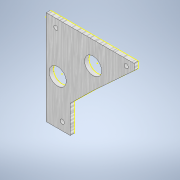
# Autodesk Inventor part: アームギアフレーム最内
Saved by Autodesk Inventor 2020.2 (Build 242310000, 310)
## iProperties
Created: 2020-02-29
Part Number: アームギアフレーム最内
Material: アルミニウム 7075
Document SubType Name: Modeling
Designer: aoyam
Density: 2.81 g/cm^3
Appearance: サテン - ブラシ仕上げ 重厚
Author: aoyam
Autodesk Inventor part; units mm, degrees
ref_plane "YZ Plane" through (0, 0, 0) normal (1, 0, 0) x (0, 1, 0)
ref_plane "XZ Plane" through (0, 0, 0) normal (0, 1, 0) x (-1, 0, 0)
sketch "ギア線図" plane through (0, 0, 0) normal (0, 0, 1) x (1, 0, 0)
  circle A0 centre (11.2246, -29.111) radius 11.1
  circle A1 centre (54.569, -27.2294) radius 20.05
  circle A2 centre (54.569, -27.2294) radius 4
  circle A3 centre (36.0807, -10.2532) radius 11.1
  circle A4 centre (39.569, -43.72) radius 2.05
  circle A5 centre (69.569, -43.72) radius 2.05
  circle A6 centre (72.4026, -13.8541) radius 2.05
  circle A7 centre (39.569, -43.72) radius 15
  circle A8 centre (69.569, -43.72) radius 15
  circle A9 centre (72.4026, -13.8541) radius 15
  circle A10 centre (54.569, -27.2294) radius 5.5 construction
  circle A11 centre (11.2246, -29.111) radius 13 construction
  circle A12 centre (54.569, -27.2294) radius 20.5 construction
  circle A13 centre (36.0807, -10.2532) radius 20.55
  circle A14 centre (36.0807, -10.2532) radius 21.5 construction
  circle A15 centre (36.0807, -10.2532) radius 13 construction
  circle A16 centre (39.569, -43.72) radius 2.5 construction
  circle A17 centre (69.569, -43.72) radius 2.5 construction
  circle A18 centre (72.4026, -13.8541) radius 2.5 construction
  circle A19 centre (11.2246, -29.111) radius 20.1
  circle A20 centre (11.2246, -29.111) radius 22 construction
  line L0 (39.569, -43.72) -> (69.569, -43.72)
  circle A21 centre (0, 0) radius 20.1
  circle A22 centre (0, 0) radius 22 construction
  circle A23 centre (39.569, -43.72) radius 9.5 construction
  circle A24 centre (69.569, -43.72) radius 9.5 construction
  circle A25 centre (72.4026, -13.8541) radius 9.5 construction
  line L1 (39.569, -43.72) -> (33.651, -38.3369)
  line L2 (39.569, -43.72) -> (54.569, -27.2294)
  circle A26 centre (33.651, -38.3369) radius 2.25
  circle A27 centre (54.569, -27.2294) radius 4.55
  point P0 (58.2233, -20.0465)
  point P1 (42.0436, -35)
  point P2 (21.5995, 15.2696)
  point P3 (38.2329, 5.9161)
  point P4 (24.1755, 8.4229)
  point P5 (21.6039, 15.1272)
  point P6 (23.3458, 16.3469)
  point P7 (23.3177, 16.3886)
  dimension "d7" = 22.2
  dimension "d8" = 40.1
  dimension "d9" = 8
  dimension "d11" = 22.2
  dimension "d12" = 4.1
  dimension "d13" = 4.1
  dimension "d14" = 4.1
  dimension "d15" = 30
  dimension "d16" = 30
  dimension "d17" = 30
  dimension "d18" = 11
  dimension "d21" = 26
  dimension "d29" = 41
  dimension "d39" = 22.2921
  dimension "d40" = 22.2921
  dimension "d41" = 22.2921
  dimension "d43" = 41.1
  dimension "d44" = 43
  dimension "d45" = 26
  dimension "d46" = 5
  dimension "d47" = 5
  dimension "d48" = 5
  dimension "d49" = 40.2
  dimension "d50" = 44
  dimension "d53" = 40.2
  dimension "d55" = 44
  dimension "d58" = 19
  dimension "d59" = 19
  dimension "d60" = 19
  dimension "d86" = 8
  dimension "d87" = 4.5
  constraints: 28 centre point, 17 coincident, 7 tangent, 6 end point, 3 concentric, 2 horizontal, 1 perpendicular, 1 other
  measures "d7" diameter of A0
  measures "d8" diameter of A1
  measures "d9" diameter of A2
  measures "d11" diameter of A3
  measures "d12" diameter of A4
  measures "d13" diameter of A5
  measures "d14" diameter of A6
  measures "d15" diameter of A7
  measures "d16" diameter of A8
  measures "d17" diameter of A9
  measures "d18" diameter of A10
  measures "d21" diameter of A11
  measures "d29" diameter of A12
  measures "d39" distance of A4.centre A1.centre
  measures "d40" distance of A5.centre A1.centre
  measures "d41" distance of A6.centre A1.centre
  measures "d43" diameter of A13
  measures "d44" diameter of A14
  measures "d45" diameter of A15
  measures "d46" diameter of A16
  measures "d47" diameter of A17
  measures "d48" diameter of A18
  measures "d49" diameter of A19
  measures "d50" diameter of A20
  measures "d53" diameter of A21
  measures "d55" diameter of A22
  measures "d58" diameter of A23
  measures "d59" diameter of A24
  measures "d60" diameter of A25
  measures "d86" distance of L1.start L1.end
  measures "d87" diameter of A26
sketch "スケッチ3" plane through (0, 0, 0) normal (0, 0, 1) x (1, 0, 0)
  circle A0 centre (54.569, -27.2294) radius 20.05 construction
  circle A1 centre (39.569, -43.72) radius 2.05 construction
  circle A2 centre (69.569, -43.72) radius 2.05 construction
  circle A3 centre (72.4026, -13.8541) radius 2.05 construction
  circle A4 centre (39.569, -43.72) radius 15 construction
  circle A5 centre (69.569, -43.72) radius 15 construction
  circle A6 centre (72.4026, -13.8541) radius 15 construction
  line L0 (39.569, -43.72) -> (45.487, -49.103)
  line L1 (45.487, -49.103) -> (39.569, -43.72)
  line L2 (39.569, -43.72) -> (33.651, -38.3369)
  line L3 (39.569, -43.72) -> (41.0777, -42.0614)
  circle A7 centre (33.651, -38.3369) radius 1.3
  circle A8 centre (45.487, -49.103) radius 1.3
  line L4 (69.569, -43.72) -> (68.0603, -42.0614)
  line L5 (69.569, -43.72) -> (75.487, -38.3369)
  line L6 (69.569, -43.72) -> (63.651, -49.103)
  circle A9 centre (63.651, -49.103) radius 1.3
  circle A10 centre (75.487, -38.3369) radius 1.3
  line L7 (72.4026, -13.8541) -> (70.609, -15.1993)
  line L8 (67.6026, -7.4541) -> (72.4026, -13.8541)
  line L9 (72.4026, -13.8541) -> (77.2027, -20.2541)
  circle A11 centre (67.6026, -7.4541) radius 1.3
  circle A12 centre (77.2027, -20.2541) radius 1.3
  circle A13 centre (39.569, -43.72) radius 5
  circle A14 centre (69.569, -43.72) radius 5
  circle A15 centre (72.4026, -13.8541) radius 5
  circle A16 centre (54.569, -27.2294) radius 4
  circle A17 centre (36.0807, -10.2532) radius 11.1 construction
  line L10 (87.4026, -58.72) -> (21.3486, -58.72)
  line L11 (87.4026, 3.1749) -> (87.4026, -58.72)
  circle A18 centre (36.0807, -10.2532) radius 6
  circle A19 centre (23.1948, 12.8161) radius 1.5
  circle A20 centre (59.3303, 1.1874) radius 1.5
  circle A21 centre (11.2246, -29.111) radius 6
  circle A22 centre (14.4482, -54.9706) radius 1.5
  line L12 (87.4026, 3.1749) -> (31.1389, 3.1749)
  line L13 (31.1389, 3.1749) -> (25.7575, 16.2256)
  line L14 (26.6296, -46.3454) -> (10.2913, -53.0824)
  line L15 (10.2913, -53.0824) -> (10.2913, -58.72)
  line L16 (10.2913, -58.72) -> (21.3486, -58.72)
  line L17 (26.6296, -46.3454) -> (26.6296, -10.2532)
  line L18 (26.6296, -10.2532) -> (18.7982, 13.9762)
  line L19 (18.7982, 13.9762) -> (25.7575, 16.2256)
  circle A23 centre (36.0807, -10.2532) radius 13 projected
  circle A24 centre (36.0807, -10.2532) radius 14
  circle A25 centre (36.0807, -10.2532) radius 17
  line L20 (50.0807, -10.2532) -> (50.0807, 3.1749)
  line L21 (26.6296, -24.2532) -> (36.0807, -24.2532)
  circle A26 centre (33.651, -38.3369) radius 2
  point P0 (0, 0)
  point P1 (0, 0)
  point P2 (30.1122, 5.6646)
  point P3 (23.0867, 0.7083)
  point P4 (26.6296, -24.3839)
  point P5 (46.5059, 3.1749)
  point P6 (40.0412, 3.1749)
  point P7 (26.6296, -20.5817)
  dimension "d61" = 8
  dimension "d62" = 8
  dimension "d63" = 2.6
  dimension "d64" = 2.6
  dimension "d65" = 8
  dimension "d66" = 8
  dimension "d67" = 2.6
  dimension "d68" = 2.6
  dimension "d69" = 8
  dimension "d70" = 8
  dimension "d71" = 2.6
  dimension "d72" = 2.6
  dimension "d73" = 10
  dimension "d74" = 10
  dimension "d75" = 10
  dimension "d76" = 8
  dimension "d79" = 12
  dimension "d82" = 26
  dimension "d83" = 1
  dimension "d84" = 3
  dimension "d85" = 4
  dimension "d98" = 12
  constraints: 44 end point, 18 centre point, 13 coincident, 8 perpendicular, 5 point on circle, 3 horizontal, 3 line through centre, 3 point on line, 2 collinear, 2 tangent, 2 vertical
  measures "d61" distance of L0.start L0.end
  measures "d62" distance of L0.start L2.end
  measures "d63" diameter of A7
  measures "d64" diameter of A8
  measures "d65" distance of L4.start L5.end
  measures "d66" distance of L4.start L6.end
  measures "d67" diameter of A9
  measures "d68" diameter of A10
  measures "d69" distance of L8.start L8.end
  measures "d70" distance of L8.end L9.end
  measures "d71" diameter of A11
  measures "d72" diameter of A12
  measures "d73" diameter of A13
  measures "d74" diameter of A14
  measures "d75" diameter of A15
  measures "d76" diameter of A16
  measures "d79" diameter of A18
  measures "d82" diameter of A23
  measures "d83" radial gap between concentric circles of A23 A24
  measures "d84" radial gap between concentric circles of A24 A25
  measures "d85" diameter of A26
  measures "d98" diameter of A21
ref_plane "作業平面1" through (0, 0, 0) normal (0, 0, -1) x (-1, 0, 0)
sketch "スケッチ9" plane through (0, 0, 0) normal (0, 0, -1) x (-1, 0, 0)
  circle A0 centre (-59.3303, 1.1874) radius 1.5 projected
  circle A1 centre (-9.9716, -0.138) radius 1.5 projected
  circle A2 centre (-14.4482, -54.9706) radius 1.5 projected
  circle A3 centre (-36.0807, -10.2532) radius 6 projected
  circle A4 centre (-11.2246, -29.111) radius 6 projected
  line L0 (-3.2194, 5.6168) -> (-3.2194, -60.6195) projected
  line L1 (-64.8213, 5.6168) -> (-3.2194, 5.6168) projected
  line L2 (-64.8213, -60.6195) -> (-64.8213, 5.6168) projected
  line L3 (-3.2194, -60.6195) -> (-64.8213, -60.6195) projected
  circle A5 centre (-14.4482, -54.9706) radius 1.5 projected
  circle A6 centre (-59.3303, 1.1874) radius 1.5 projected
  line L4 (-20.0136, -60.6195) -> (-20.0136, -41.0239)
  line L5 (-20.0136, -41.0239) -> (-36.0807, -25.2636)
  line L6 (-36.0807, -25.2636) -> (-64.8213, 1.2001)
  line L7 (-59.3303, 1.1874) -> (-52.604, 1.362)
  point P0 (0, 0)
  dimension "d104" = 28
  dimension "d106" = 29
  constraints: 8 end point, 2 point on line, 1 vertical, 4 other
  measures "d104" distance of A3.centre A1.centre
  measures "d106" distance of A4.centre A1.centre
extrude "押し出し8" add sketch "スケッチ9" along normal blind 3 contours L0 L3 L4 L5 L6 L2 L1
sketch "スケッチ10" plane through (0, 0, -3) normal (0, 0, -1) x (-1, 0, 0)
  line L0 (-20.0136, -60.6195) -> (-3.2194, -60.6195) projected
  line L1 (-3.2194, -60.6195) -> (-3.2194, 5.6168) projected
  line L2 (-3.2194, 5.6168) -> (-64.8213, 5.6168) projected
  line L3 (-64.8213, 5.6168) -> (-64.8213, 1.2001) projected
  line L4 (-64.8213, 1.2001) -> (-36.0807, -25.2636) projected
  line L5 (-36.0807, -25.2636) -> (-20.0136, -41.0239) projected
  line L6 (-20.0136, -41.0239) -> (-20.0136, -60.6195) projected
  circle A0 centre (-59.3303, 1.1874) radius 1.5 projected
  circle A1 centre (-9.9716, -0.138) radius 1.5 projected
  circle A2 centre (-14.4482, -54.9706) radius 1.5 projected
  circle A3 centre (-11.2246, -29.111) radius 6 projected
  circle A4 centre (-36.0807, -10.2532) radius 6 projected
  point P0 (0, 0)
equation "\"d40\" = d39"
equation "\"d41\" = d40"
